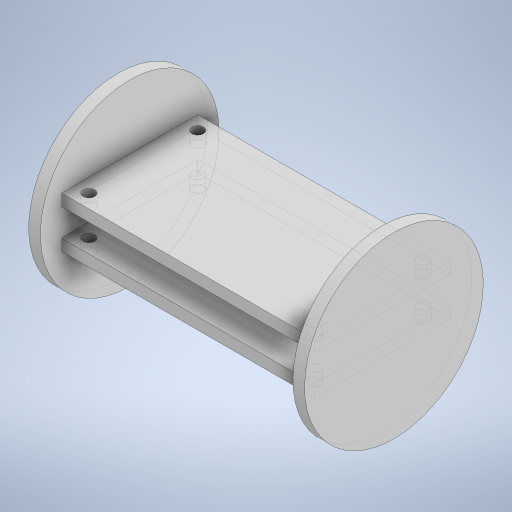
# Autodesk Inventor part: koszyk na elektro
Saved by Autodesk Inventor 2023.2 (Build 272271000, 271)
## iProperties
Created: 2022-12-20
Part Number: koszyk na elektro
Material: Generic
Document SubType Name: Modeling
Designer: Admin
Density: 1 g/cm^3
Appearance: Default
Author: Admin
Autodesk Inventor part; units mm, degrees
sketch "Sketch2" plane through (0, 0, 0) normal (0, 1, 0) x (-1, 0, 0)
  line L0 (0, 0) -> (65, 0)
  line L1 (65, 0) -> (65, -35)
  line L2 (65, -35) -> (0, -35)
  line L3 (0, -35) -> (0, 0)
  dimension "d1" = 65
  dimension "d2" = 35
  constraints: 8 end point, 2 parallel, 1 horizontal, 1 perpendicular
  measures "d1" distance of L1.end L2.end
  measures "d2" distance of L0.end L1.end
extrude "Extrusion1" add sketch "Sketch2" along normal blind 3
ref_plane "Work Plane1" through (0, 1.5, 0) normal (0, 1, 0) x (-1, 0, 0)
sketch "Sketch5" plane through (0, 0, 0) normal (0, 1, 0) x (-1, 0, 0)
  circle A0 centre (3.5, -31.5) radius 1.5
  circle A1 centre (3.5, -3.5) radius 1.5
  circle A2 centre (61.5, -31.5) radius 1.5
  circle A3 centre (61.5, -3.5) radius 1.5
  line L0 (0, 0) -> (0, -35) projected
  line L1 (65, -35) -> (65, 0) projected
  line L2 (0, -35) -> (65, -35) projected
  line L3 (65, 0) -> (0, 0) projected
  dimension "d22" = 3
  dimension "d23" = 3
  dimension "d24" = 3
  dimension "d25" = 3
  dimension "d26" = 3.5
  dimension "d27" = 3.5
  dimension "d28" = 3.5
  dimension "d29" = 3.5
  dimension "d30" = 3.5
  dimension "d31" = 3.5
  dimension "d32" = 3.5
  dimension "d33" = 3.5
  constraints: 4 centre point
  measures "d22" diameter of A0
  measures "d23" diameter of A1
  measures "d24" diameter of A2
  measures "d25" diameter of A3
  measures "d26" distance from line of L0 A0.centre
  measures "d27" distance from line of L1 A2.centre
  measures "d28" distance from line of L2 A2.centre
  measures "d29" distance from line of L2 A0.centre
  measures "d30" distance from line of L3 A3.centre
  measures "d31" distance from line of L1 A3.centre
  measures "d32" distance from line of L0 A1.centre
  measures "d33" distance from line of L3 A1.centre
extrude "Extrusion4" cut sketch "Sketch5" along normal blind 10 contours A0 | A1 | A2 | A3
pattern_linear "Rectangular Pattern1" count 2 spacing 10 along (0, -1, 0)
ref_plane "Work Plane2" through (-65, -7, 0) normal (1, 0, 0) x (0, 1, 0)
sketch "Sketch6" plane through (-65, -7, 0) normal (1, 0, 0) x (0, 1, 0)
  line L0 (7, -35) -> (10, -35) projected
  line L1 (-3, -35) -> (0, -35) projected
  line L2 (-3, 0) -> (0, 0) projected
  circle A0 centre (3.5, -17.5) radius 23
  line L3 (-3, -35) -> (-3, 0) projected
  line L4 (10, -35) -> (10, 0) projected
  point P0 (7, 0)
  point P1 (8.5, -35)
  point P2 (-1.5, -35)
  point P3 (-1.5, 0)
  point P4 (-1.5, -35)
  constraints: 4 midpoint, 1 centre point
extrude "Extrusion5" add sketch "Sketch6" against normal blind 3
ref_plane "Work Plane3" through (0, 0, 0) normal (1, 0, 0) x (0, 1, 0)
sketch "Sketch7" plane through (0, 0, 0) normal (1, 0, 0) x (0, 1, 0)
  circle A0 centre (-3.5, -17.5) radius 23
  line L0 (-10, 0) -> (-10, -35) projected
  line L1 (3, 0) -> (3, -35) projected
  line L2 (0, 0) -> (3, 0) projected
  line L3 (-10, -35) -> (-7, -35) projected
  dimension "d49" = 46
  constraints: 1 centre point
  measures "d49" diameter of A0
extrude "Extrusion6" add sketch "Sketch7" along normal blind 3
equation "\"d26\" = d27"
equation "\"d29\" = d28"
equation "\"d30\" = d28"
equation "\"d31\" = d27"
equation "\"d32\" = d26"
equation "\"d33\" = d30"
body "Solid1"
